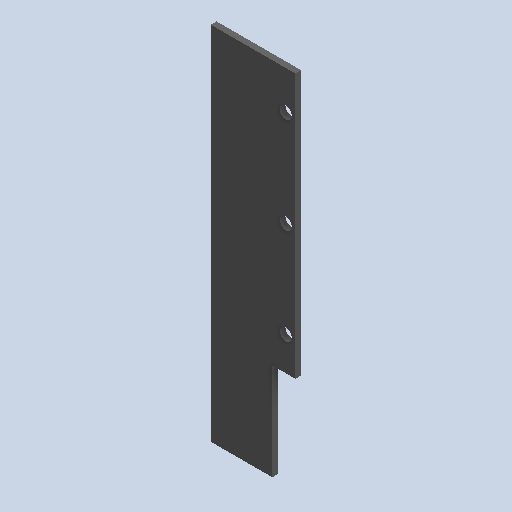
# Autodesk Inventor part: rail_backcover
Saved by Autodesk Inventor 2024.1 (Build 281209000, 209)
## iProperties
Created: 2025-01-18
Part Number: rail_backcover
Material: 一般
Document SubType Name: Modeling
Designer: hibik
Density: 1 g/cm^3
Appearance: 既定
Author: hibik
Autodesk Inventor part; units mm, degrees
ref_plane "YZ Plane" through (0, 0, 0) normal (1, 0, 0) x (0, 1, 0)
ref_plane "XZ Plane" through (0, 0, 0) normal (0, 1, 0) x (-1, 0, 0)
ref_plane "XY Plane" through (0, 0, 0) normal (0, 0, 1) x (1, 0, 0)
sketch "スケッチ1" plane through (0, 0, 0) normal (0, 0, 1) x (1, 0, 0)
  line L0 (0, 0) -> (-22, 0)
  line L1 (-22, 0) -> (-22, 94)
  line L2 (-22, 94) -> (0, 94)
  line L3 (0, 94) -> (0, 0)
  dimension "d0" = 22
  dimension "d1" = 94
  constraints: 8 end point, 2 parallel, 1 horizontal, 1 perpendicular
  measures "d0" distance of L1.end L2.end
  measures "d1" distance of L0.end L1.end
extrude "押し出し1" add sketch "スケッチ1" along normal blind 1.5
sketch "スケッチ2" plane through (0, 0, 0) normal (0, 0, -1) x (-1, 0, 0)
  line L0 (5, 24.2) -> (5, 94) projected
  circle A0 centre (2.5, 84) radius 1.6
  line L1 (0, 94) -> (22, 94) projected
  line L2 (5, 94) -> (0, 94)
  circle A1 centre (2.5, 59) radius 1.6
  circle A2 centre (2.5, 34) radius 1.6
  circle A3 centre (2.5, 9) radius 1.6
  point P0 (0, 0)
  point P1 (2.5, 94)
  dimension "d4" = 3.2
  dimension "d5" = 10
  dimension "d8" = 25
  constraints: 4 centre point, 2 end point, 1 collinear, 1 midpoint, 1 vertical, 1 vertical alignment, 6 other
  measures "d4" diameter of A0
  measures "d5" distance from line of L1 A0.centre
  measures "d8" distance of A0.centre A1.centre
extrude "押し出し2" cut sketch "スケッチ2" against normal through all
sketch "スケッチ3" plane through (0, 0, 0) normal (0, 0, -1) x (-1, 0, 0)
  line L0 (3.2909, 24.2) -> (5, 24.2) projected
  line L1 (0, 0) -> (0, 94) projected
  line L2 (0, 25.2) -> (6, 25.2)
  line L3 (6, 25.2) -> (6, 0)
  line L4 (6, 0) -> (0, 0)
  line L5 (0, 0) -> (0, 25.2)
  line L6 (5, 14.2) -> (5, 24.2) projected
  line L7 (22, 0) -> (0, 0) projected
  dimension "d15" = 1
  dimension "d16" = 1
  constraints: 8 end point, 2 parallel, 1 collinear, 1 horizontal, 1 perpendicular, 1 point on line
  measures "d15" distance between parallel lines of L2 L0
  measures "d16" distance between parallel lines of L3 L6
extrude "押し出し3" cut sketch "スケッチ3" against normal through all
